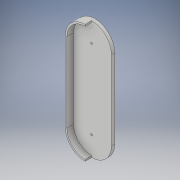
# Autodesk Inventor part: ChainGuard
Saved by Autodesk Inventor 2017 (Build 210142000, 142)
## iProperties
Created: 2017-11-28
Part Number: ChainGuard
Material: Generic
Document SubType Name: Modeling
Designer: User
Density: 1 g/cm^3
Appearance: Default
Author: User
Autodesk Inventor part; units mm, degrees
ref_plane "YZ Plane" through (0, 0, 0) normal (1, 0, 0) x (0, 1, 0)
ref_plane "XZ Plane" through (0, 0, 0) normal (0, 1, 0) x (-1, 0, 0)
ref_plane "XY Plane" through (0, 0, 0) normal (0, 0, 1) x (1, 0, 0)
sketch "Sketch1" plane through (0, 0, 0) normal (0, 0, 1) x (1, 0, 0)
  line L0 (0, 0) -> (0, -152.4)
  line L1 (76.2, -152.4) -> (76.2, 0)
  arc A0 (0, -152.4) -> (76.2, -152.4) centre (38.1, -152.4) ccw
  arc A1 (76.2, 0) -> (0, 0) centre (38.1, 0) ccw
  circle A2 centre (38.1, 0) radius 1.5875
  circle A3 centre (38.1, -152.4) radius 1.5875
  dimension "d17" = 3.175
  dimension "d18" = 3.175
  constraints: 4 centre point, 4 end point, 4 point on circle, 2 coincident, 1 vertical
  measures "d17" diameter of A2
  measures "d18" diameter of A3
extrude "Extrusion1" add sketch "Sketch1" along normal blind 6.35 contours A1 L1 A0 L0 | A2 | A3
extrude "Extrusion4" cut sketch "Sketch1" along normal blind 12.7 contours A2 | A3
sketch "Sketch3" plane through (0, 0, 6.35) normal (0, 0, 1) x (1, 0, 0)
  arc A0 (0, -152.4) -> (76.2, -152.4) centre (38.1, -152.4) ccw projected
  line L0 (38.1, -190.5) -> (38.1, -187.325)
  arc A1 (3.175, -152.4) -> (38.1, -187.325) centre (38.1, -152.4) ccw
  arc A2 (76.2, 0) -> (0, 0) centre (38.1, 0) ccw projected
  line L1 (38.1, 38.1) -> (38.1, 34.925)
  arc A3 (38.1, 34.925) -> (3.175, 0) centre (38.1, 0) ccw
  line L2 (3.175, -152.4) -> (3.175, 0)
  line L3 (0, 0) -> (0, -152.4) projected
  dimension "d21" = 3.175
  dimension "d23" = 3.175
  dimension "d24" = 3.175
  constraints: 6 end point, 6 point on circle, 2 centre point, 2 concentric, 2 vertical
  measures "d21" distance of L0.start L0.end
  measures "d23" distance of L1.start L1.end
  measures "d24" distance of L3.start L2.end
extrude "Extrusion5" add sketch "Sketch3" along normal blind 12.7
sketch "Sketch4" plane through (0, 0, 6.35) normal (0, 0, 1) x (1, 0, 0)
  point P0 (0, 0)
body "Solid1"
